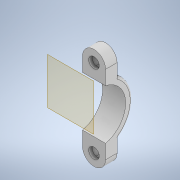
# Autodesk Inventor part: Bracket22_2
Saved by Autodesk Inventor 2020 (Build 240168000, 168)
## iProperties
Created: 2020-05-20
Part Number: Bracket22_2
Material: Generisch
Document SubType Name: Modeling
Designer: hpcwoess
Density: 1 g/cm^3
Appearance: Vorgabe
Author: hpcwoess
Autodesk Inventor part; units mm, degrees
ref_plane "YZ Plane" through (0, 0, 0) normal (1, 0, 0) x (0, 1, 0)
ref_plane "XZ Plane" through (0, 0, 0) normal (0, 1, 0) x (-1, 0, 0)
ref_plane "Arbeitsebene1" through (0, 0, -17.5) normal (0, 0, 1) x (1, 0, 0)
sketch "Skizze1" plane through (0, 0, -17.5) normal (0, 0, 1) x (1, 0, 0)
  arc A0 (5.2, -17) -> (15.2, -17) centre (10.2, -17) ccw
  circle A1 centre (10.2, -17) radius 2.3
  circle A2 centre (10.2, 17) radius 2.3
  arc A3 (15.2, 17) -> (5.2, 17) centre (10.2, 17) ccw
  line L0 (15.2, 17) -> (15.2, -17)
  line L1 (5.2, -17) -> (5.2, 17)
  point P0 (0, 0)
  dimension "d17" = 34
  dimension "d19" = 5
  dimension "d20" = 5
  dimension "d21" = 4.6
  dimension "d22" = 4.6
  dimension "d23" = 5.2
  dimension "d24" = 15.2
  dimension "d25" = 17
  constraints: 4 centre point, 4 end point, 4 point on circle, 2 coincident, 2 vertical
  measures "d17" distance of A0.centre A2.centre
  measures "d19" radius of A3
  measures "d20" radius of A0
  measures "d21" diameter of A2
  measures "d22" diameter of A1
  measures "d23" distance from line of L1 point (0, 0)
  measures "d24" distance from line of L0 point (0, 0)
  measures "d25" vertical distance of A0.centre point (0, 0)
extrude "Extrusion1" add sketch "Skizze1" against normal blind 15
sketch "Skizze2" plane through (15.2, -17, -17.5) normal (1, 0, 0) x (0, 0, -1)
  circle A0 centre (-2.4, 17) radius 11.1
  circle A1 centre (-2.4, 17) radius 14.1
  line L0 (0, 39) -> (15, 39) projected
  line L1 (5, 39) -> (5, 29.0021)
  line L2 (5, 39) -> (-2.0976, 39.0148)
  line L3 (-2.0976, 39.0148) -> (-4.3191, 38.5001)
  line L4 (-4.3191, 38.5001) -> (-4.8354, 27.8295)
  line L5 (-4.8906, 6.183) -> (-12.1302, -16.582)
  line L6 (-12.1302, -16.582) -> (7.7221, -22.1422)
  line L7 (7.7221, -22.1422) -> (5, -5)
  line L8 (0, -5) -> (15, -5) projected
  line L9 (5, -5) -> (5, 4.9979)
  line L10 (0, 0) -> (0, -5) projected
  line L11 (36.0228, 70.8555) -> (-22.3921, 70.8555)
  line L12 (-22.3921, 70.8555) -> (-22.3921, -28.3632)
  line L13 (-22.3921, -28.3632) -> (36.0228, -28.3632)
  line L14 (36.0228, -28.3632) -> (36.0228, 70.8555)
  point P0 (-17.5, 17)
  point P1 (-5.8022, 3.3166)
  point P2 (-4.6862, 30.9134)
  dimension "d5" = 3
  dimension "d6" = 5
  dimension "d26" = 44
  dimension "d27" = 22
  dimension "d28" = 22.2
  dimension "d29" = 15.1
  constraints: 24 end point, 4 point on circle, 4 point on line, 2 centre point, 2 parallel, 2 perpendicular, 1 horizontal
  measures "d5" radial gap between concentric circles of A0 A1
  measures "d6" distance between parallel lines of L9 L10
  measures "d26" distance between parallel lines of L0 L8
  measures "d27" distance from line of A0.centre L0
  measures "d28" diameter of A0
  measures "d29" distance of point (-17.5, 17) A0.centre
extrude "Extrusion2" cut sketch "Skizze2" against normal blind 10 contours A0 | L14 L13 L12 L11
sketch "Skizze3" plane through (15.2, -17, -22.5) normal (0, 0, -1) x (-1, 0, 0)
  circle A0 centre (5, 34) radius 2.3 projected
  line L0 (2.8638, 30.3) -> (0.7276, 34)
  line L1 (0.7276, 34) -> (2.8638, 37.7)
  line L2 (2.8638, 37.7) -> (7.1362, 37.7)
  line L3 (7.1362, 37.7) -> (9.2724, 34)
  line L4 (9.2724, 34) -> (7.1362, 30.3)
  line L5 (7.1362, 30.3) -> (2.8638, 30.3)
  line L6 (0.7276, 0) -> (2.8638, 3.7)
  line L7 (2.8638, 3.7) -> (7.1362, 3.7)
  line L8 (7.1362, 3.7) -> (9.2724, 0)
  line L9 (9.2724, 0) -> (7.1362, -3.7)
  line L10 (7.1362, -3.7) -> (2.8638, -3.7)
  line L11 (2.8638, -3.7) -> (0.7276, 0)
  point P0 (15.2, 17)
  point P1 (5, 34)
  point P2 (5, 0)
  point P3 (5, 0)
  point P4 (5.6446, 34.7922)
  point P5 (4.3554, 34.7922)
  dimension "d9" = 7.4
  dimension "d10" = 7.4
  constraints: 24 end point, 2 coincident, 2 horizontal, 27 other
  measures "d9" distance between parallel lines of L0 L3
  measures "d10" distance between parallel lines of L11 L8
extrude "Extrusion3" cut sketch "Skizze3" along normal blind 10 and the other way blind 3.5 contours A0 | L0 L1 L2 L3 L4 L5 | L6 L7 L8 L9 L10 L11
fillet "Rundung1" radius 1 2 edges at (15.2, 0, -29.2) (5.2, 0, -29.2)
equation "\"d20\" = d19"
equation "\"d27\" = 0.5 * d26"
equation "\"d10\" = d9"
